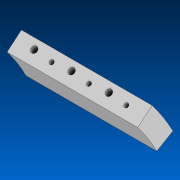
# Autodesk Inventor part: HoodBraceExtension
Saved by Autodesk Inventor 2022 (Build 260153000, 153)
## iProperties
Created: 2022-04-24
Part Number: HoodBraceExtension
Material: Generic
Document SubType Name: Modeling
Designer: omard
Density: 1 g/cm^3
Appearance: Default
Author: omard
Autodesk Inventor part; units mm, degrees
ref_plane "YZ Plane" through (0, 0, 0) normal (1, 0, 0) x (0, 1, 0)
ref_plane "XZ Plane" through (0, 0, 0) normal (0, 1, 0) x (-1, 0, 0)
sketch "Sketch1" plane through (0, 0, 0) normal (1, 0, 0) x (0, 1, 0)
  arc A0 (0, -277.0467) -> (178.0822, -212.2301) centre (0, 0) ccw
  arc A1 (0, -302.4467) -> (194.409, -231.6876) centre (0, 0) ccw
  line L0 (178.0822, -212.2301) -> (194.409, -231.6876)
  line L1 (0, -277.0467) -> (0, -302.4467)
  line L2 (168.1662, -220.1704) -> (184.6802, -239.851)
  line L3 (184.6802, -239.851) -> (204.1378, -223.5242)
  line L4 (204.1378, -223.5242) -> (187.811, -204.0667)
  line L5 (187.811, -204.0667) -> (168.3534, -220.3935)
  line L6 (168.3534, -220.3935) -> (204.1378, -223.5242) construction
  line L7 (184.6802, -239.851) -> (187.811, -204.0667) construction
  arc A2 (0, -277.0467) -> (138.5234, -239.9295) centre (0, 0) ccw
  line L8 (138.5234, -239.9295) -> (151.2234, -261.9266)
  line L9 (162.2219, -255.5766) -> (140.2248, -268.2766)
  line L10 (140.2248, -268.2766) -> (127.3792, -246.0273)
  line L11 (127.5248, -246.2795) -> (149.5219, -233.5795)
  line L12 (149.5219, -233.5795) -> (162.2219, -255.5766)
  line L13 (162.2219, -255.5766) -> (127.5248, -246.2795) construction
  line L14 (140.2248, -268.2766) -> (149.5219, -233.5795) construction
  point P0 (186.2456, -221.9589)
  point P1 (184.5088, -239.6467)
  point P2 (144.8734, -250.928)
  point P3 (140.0915, -268.0455)
  dimension "d1" = 277.0467
  dimension "d2" = 40
  dimension "d4" = 25.4
  dimension "d5" = 25.4
  dimension "d32" = 30
  dimension "d33" = 25.4
  constraints: 30 end point, 10 point on circle, 7 midpoint, 5 parallel, 4 point on line, 3 centre point, 3 coincident, 3 perpendicular, 2 line through centre, 1 concentric, 1 tangent, 1 vertical
  measures "d1" radius of A0
  measures "d2" angle of L1 L0
  measures "d4" distance of L3.end L2.end
  measures "d5" distance of L1.start L1.end
  measures "d33" distance between parallel lines of L10 L12
extrude "Extrusion1" add sketch "Sketch1" along normal mid plane 177.8 contours A0 L11 L10 | L11 L12 A1 L8 | L8 A1 L10 L11 | A0 L2 A1 L12 L11
sketch "Sketch3" plane through (-88.9, 168.1662, -220.1704) normal (0, 0.7660444, 0.6427876) x (1, 0, 0)
  line L0 (88.9, 0) -> (88.9, 25.6912) projected
  line L1 (177.8, 25.4245) -> (177.8, 0) projected
  point P0 (88.9, -276.7555)
  point P1 (152.4, 12.9912)
  dimension "d17" = 25.4
  dimension "d18" = 12.7
  measures "d17" distance from line of point (152.4, 12.991) L1
  measures "d18" vertical distance of L0.end point (152.4, 12.991)
hole "Hole2" at (63.5, 176.5168, -230.1223) direction (0, -0.7660444, -0.6427876) diameter 4.445 depth 38.1 counterbore diameter 5.588 counterbore depth 8.255
pattern_linear "Rectangular Pattern2" count 3 spacing 50.8 along (-1, 0, 0) of "Hole2"
sketch "Sketch5" plane through (-88.9, 140.2248, -268.2766) normal (0, -0.8660254, -0.5) x (1, 0, 0)
  point P0 (88.9, 302.4467)
sketch "Sketch6" plane through (-88.9, 140.2248, -268.2766) normal (0, -0.8660254, -0.5) x (1, 0, 0)
  line L0 (0, 0.2668) -> (0, 25.6912) projected
  line L1 (0, 25.6912) -> (177.8, 25.6912) projected
  point P0 (88.9, 302.4467)
  point P1 (25.4, 12.7)
  dimension "d50" = 25.4
  dimension "d51" = 12.9912
  measures "d50" distance from line of L0 point (25.4, 12.7)
  measures "d51" distance from line of L1 point (25.4, 12.7)
hole "Hole3" at (-63.5, 133.8748, -257.278) direction (0, 0.8660254, 0.5) diameter 4.445 end through all
ref_plane "Work Plane1" through (-88.9, 162.0885, -255.3455) normal (0, -0.8660254, -0.5) x (1, 0, 0)
sketch "Sketch7" plane through (-88.9, 162.0885, -255.3455) normal (0, -0.8660254, -0.5) x (1, 0, 0)
  circle A0 centre (25.4, 12.4332) radius 2.2225 projected
  circle A1 centre (25.4, 12.4332) radius 4.064
  point P0 (88.9, 302.18)
  dimension "d44" = 8.128
  constraints: 1 centre point, 1 coincident
  measures "d44" diameter of A1
extrude "Extrusion2" cut sketch "Sketch7" against normal through all contours A0 | A1
pattern_linear "Rectangular Pattern3" count 3 spacing 50.8 along (1, 0, 0) of "Extrusion2", "Hole3"
body "Solid1"
